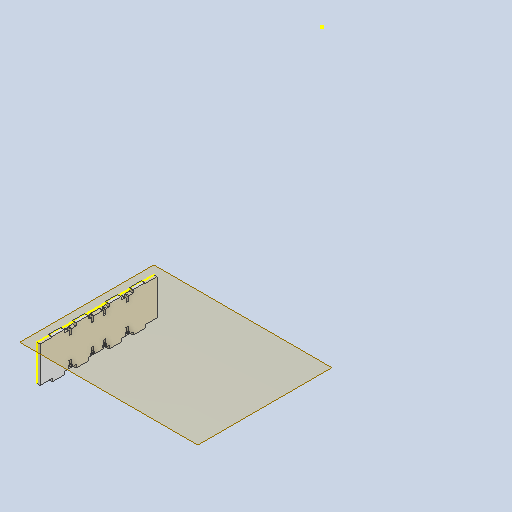
# Autodesk Inventor part: стенка
Saved by Autodesk Inventor 2024.2 (Build 282272000, 272)
## iProperties
Created: 2025-12-09
Part Number: стенка
Material: Типовые
Document SubType Name: Modeling
Designer: katya_notebook
Mass: 65.1748 g
Surface Area: 247.334 cm^2
Volume: 65.1748 cm^3
Density: 1 g/cm^3
Appearance: По умолчанию
Author: katya_notebook
Autodesk Inventor part; units mm, degrees
ref_plane "YZ Plane" through (0, 0, 0) normal (1, 0, 0) x (0, 1, 0)
ref_plane "XZ Plane" through (0, 0, 0) normal (0, 1, 0) x (-1, 0, 0)
ref_plane "XY Plane" through (0, 0, 0) normal (0, 0, 1) x (1, 0, 0)
ref_plane "РабПлоскость1" through (-475.2675, -216.9886, 379.0883) normal (0, 1, 0) x (-1, 0, 0)
sketch "Эскиз1" plane through (-475.2675, -216.9886, 379.0883) normal (0, 1, 0) x (-1, 0, 0)
  line L0 (135, 97.5) -> (129, 97.5)
  line L1 (129, 97.5) -> (129, -97.5)
  line L2 (129, -97.5) -> (135, -97.5)
  line L3 (135, -97.5) -> (135, 97.5)
  line L4 (135, -97.5) -> (135, 97.5) projected
  line L5 (127, 97.5) -> (62.5237, 97.5) projected
  line L6 (62.5237, -97.5) -> (127, -97.5) projected
  point P0 (-475.2675, -379.0883)
  dimension "d0" = 0
  dimension "d1" = 6
  dimension "d2" = 0
  dimension "d3" = 0
  constraints: 8 end point, 2 parallel, 1 horizontal, 1 perpendicular, 1 vertical alignment
  measures "d0" horizontal extent of L3
  measures "d1" distance of L0.start L0.end
  measures "d2" distance between parallel lines of L6 L2
  measures "d3" distance between parallel lines of L0 L5
ref_plane "РабПлоскость2" through (-610.2675, -276.6936, 277.5883) normal (0, 1, 0) x (0, 0, 1)
extrude "Выдавливание1" add sketch "Эскиз1" against normal up to surface (59.705 mm away)
sketch "Эскиз2" plane through (-610.2675, -216.9886, 281.5883) normal (-1, 0, 0) x (0, 0, 1)
  line L0 (175, -4) -> (187, -4) projected
  line L1 (195, 0) -> (195, -59.705) projected
  line L2 (0, 0) -> (195, 0) projected
  line L3 (0, 0) -> (0, -59.705) projected
  point P0 (-281.5883, 216.9886)
  point P1 (195, -59.705)
  point P2 (0, -59.705)
  constraints: 2 other
sketch "Эскиз3" plane through (-610.2675, -276.6936, 281.5883) normal (-1, 0, 0) x (0, 0, 1)
  line L0 (195, 0) -> (0, 0) projected
  line L1 (175, 0) -> (155, 0)
  line L2 (155, 0) -> (155, -5)
  line L3 (155, -5) -> (175, -5)
  line L4 (175, -5) -> (175, 0)
  line L5 (195, 59.705) -> (195, 0) projected
  line L6 (135, 0) -> (115, 0)
  line L7 (115, 0) -> (115, -5)
  line L8 (115, -5) -> (135, -5)
  line L9 (135, -5) -> (135, 0)
  line L10 (20, 0) -> (40, 0)
  line L11 (40, 0) -> (40, -5)
  line L12 (40, -5) -> (20, -5)
  line L13 (20, -5) -> (20, 0)
  line L14 (60, 0) -> (80, 0)
  line L15 (80, 0) -> (80, -5)
  line L16 (80, -5) -> (60, -5)
  line L17 (60, -5) -> (60, 0)
  line L18 (97.5, 27.8525) -> (226.4185, 27.8525)
  line L19 (195, 55.705) -> (0, 55.705)
  line L20 (175, 55.705) -> (155, 55.705)
  line L21 (155, 55.705) -> (155, 60.705)
  line L22 (155, 60.705) -> (175, 60.705)
  line L23 (175, 60.705) -> (175, 55.705)
  line L24 (135, 55.705) -> (115, 55.705)
  line L25 (115, 55.705) -> (115, 60.705)
  line L26 (115, 60.705) -> (135, 60.705)
  line L27 (135, 60.705) -> (135, 55.705)
  line L28 (20, 55.705) -> (40, 55.705)
  line L29 (40, 55.705) -> (40, 60.705)
  line L30 (40, 60.705) -> (20, 60.705)
  line L31 (20, 60.705) -> (20, 55.705)
  line L32 (60, 55.705) -> (80, 55.705)
  line L33 (80, 55.705) -> (80, 60.705)
  line L34 (80, 60.705) -> (60, 60.705)
  line L35 (60, 60.705) -> (60, 55.705)
  point P0 (-281.5883, 276.6936)
  point P1 (40, 55.705)
  point P2 (80, 55.705)
  point P3 (40, 0)
  point P4 (80, 0)
  point P5 (115, 55.705)
  point P6 (155, 55.705)
  point P7 (115, 0)
  point P8 (155, 0)
  dimension "d8" = 5
  dimension "d9" = 20
  dimension "d10" = 20
  dimension "d11" = 20
  dimension "d12" = 20
  dimension "d13" = 5
  dimension "d14" = 20
  dimension "d15" = 20
  dimension "d16" = 20
  dimension "d17" = 20
  dimension "d43" = 5
  constraints: 68 end point, 17 symmetric about line, 8 parallel, 8 point on line, 5 horizontal, 4 perpendicular
  measures "d8" distance of L3.end L1.start
  measures "d9" distance of L2.end L3.end
  measures "d10" distance of L0.start L1.start
  measures "d11" distance of L7.end L8.end
  measures "d12" distance of L1.end L6.start
  measures "d13" distance of L10.end L11.end
  measures "d14" distance of L11.end L12.end
  measures "d15" distance of L10.start L0.end
  measures "d16" distance of L15.end L16.end
  measures "d17" distance of L14.start L10.end
  measures "d43" distance of L16.end L14.start
extrude "Выдавливание3" add sketch "Эскиз3" against normal blind 6
sketch "Эскиз4" plane through (-610.2675, -276.6936, 281.5883) normal (-1, 0, 0) x (0, 0, 1)
  point P0 (-281.5883, 276.6936)
sketch "Эскиз5" plane through (-610.2675, -276.6936, 281.5883) normal (-1, 0, 0) x (0, 0, 1)
  point P0 (-281.5883, 276.6936)
sketch "Эскиз6" plane through (-610.2675, -276.6936, 281.5883) normal (-1, 0, 0) x (0, 0, 1)
  line L0 (111.125, 1.5) -> (104.625, 1.5)
  line L1 (104.625, 1.5) -> (104.625, 4.5)
  line L2 (104.625, 4.5) -> (111.125, 4.5)
  line L3 (111.125, 4.5) -> (111.125, 1.5)
  line L4 (115, 0) -> (115, -5) projected
  line L5 (90.375, 1.5) -> (83.875, 1.5)
  line L6 (83.875, 1.5) -> (83.875, 4.5)
  line L7 (83.875, 4.5) -> (90.375, 4.5)
  line L8 (90.375, 4.5) -> (90.375, 1.5)
  line L9 (111.125, 3) -> (104.625, 3)
  line L10 (115, 0) -> (80, 0) projected
  line L11 (106.125, 6) -> (109.625, 6)
  line L12 (109.625, 6) -> (109.625, 0)
  line L13 (109.625, 0) -> (106.125, 0)
  line L14 (106.125, 0) -> (106.125, 6)
  line L15 (106.125, 6) -> (109.625, 0) construction
  line L16 (109.625, 6) -> (106.125, 0) construction
  line L17 (90.375, 3) -> (83.875, 3)
  line L18 (87.125, 1.5) -> (87.125, 4.5)
  line L19 (85.375, 6) -> (88.875, 6)
  line L20 (88.875, 6) -> (88.875, 0)
  line L21 (88.875, 0) -> (85.375, 0)
  line L22 (85.375, 0) -> (85.375, 6)
  line L23 (85.375, 6) -> (88.875, 0) construction
  line L24 (88.875, 6) -> (85.375, 0) construction
  line L25 (148.25, 1.5) -> (141.75, 1.5)
  line L26 (141.75, 1.5) -> (141.75, 4.5)
  line L27 (141.75, 4.5) -> (148.25, 4.5)
  line L28 (148.25, 4.5) -> (148.25, 1.5)
  line L29 (148.25, 3) -> (141.75, 3)
  line L30 (143.25, 12) -> (146.75, 12)
  line L31 (146.75, 12) -> (146.75, -6)
  line L32 (146.75, -6) -> (143.25, -6)
  line L33 (143.25, -6) -> (143.25, 12)
  line L34 (143.25, 12) -> (146.75, -6) construction
  line L35 (146.75, 12) -> (143.25, -6) construction
  line L36 (155, 0) -> (155, -5) projected
  line L37 (53.25, 1.5) -> (46.75, 1.5)
  line L38 (46.75, 1.5) -> (46.75, 4.5)
  line L39 (46.75, 4.5) -> (53.25, 4.5)
  line L40 (53.25, 4.5) -> (53.25, 1.5)
  line L41 (53.25, 3) -> (46.75, 3)
  line L42 (48.25, 12) -> (51.75, 12)
  line L43 (51.75, 12) -> (51.75, -6)
  line L44 (51.75, -6) -> (48.25, -6)
  line L45 (48.25, -6) -> (48.25, 12)
  line L46 (48.25, 12) -> (51.75, -6) construction
  line L47 (51.75, 12) -> (48.25, -6) construction
  line L48 (60, 0) -> (60, -5) projected
  line L49 (195, 59.705) -> (195, 0) projected
  line L50 (195, 29.8525) -> (88.875, 29.8525)
  line L51 (111.125, 58.205) -> (104.625, 58.205)
  line L52 (104.625, 58.205) -> (104.625, 55.205)
  line L53 (104.625, 55.205) -> (111.125, 55.205)
  line L54 (111.125, 55.205) -> (111.125, 58.205)
  line L55 (115, 59.705) -> (115, 64.705)
  line L56 (90.375, 58.205) -> (83.875, 58.205)
  line L57 (83.875, 58.205) -> (83.875, 55.205)
  line L58 (83.875, 55.205) -> (90.375, 55.205)
  line L59 (90.375, 55.205) -> (90.375, 58.205)
  line L60 (111.125, 56.705) -> (104.625, 56.705)
  line L61 (115, 59.705) -> (80, 59.705)
  line L62 (106.125, 53.705) -> (109.625, 53.705)
  line L63 (109.625, 53.705) -> (109.625, 59.705)
  line L64 (109.625, 59.705) -> (106.125, 59.705)
  line L65 (106.125, 59.705) -> (106.125, 53.705)
  line L66 (106.125, 53.705) -> (109.625, 59.705) construction
  line L67 (109.625, 53.705) -> (106.125, 59.705) construction
  line L68 (90.375, 56.705) -> (83.875, 56.705)
  line L69 (87.125, 58.205) -> (87.125, 55.205)
  line L70 (85.375, 53.705) -> (88.875, 53.705)
  line L71 (88.875, 53.705) -> (88.875, 59.705)
  line L72 (88.875, 59.705) -> (85.375, 59.705)
  line L73 (85.375, 59.705) -> (85.375, 53.705)
  line L74 (85.375, 53.705) -> (88.875, 59.705) construction
  line L75 (88.875, 53.705) -> (85.375, 59.705) construction
  line L76 (146.75, 65.705) -> (143.25, 65.705)
  line L77 (146.75, 47.705) -> (146.75, 65.705)
  line L78 (146.75, 47.705) -> (143.25, 65.705) construction
  line L79 (143.25, 47.705) -> (146.75, 65.705) construction
  line L80 (143.25, 65.705) -> (143.25, 47.705)
  line L81 (141.75, 58.205) -> (141.75, 55.205)
  line L82 (148.25, 58.205) -> (141.75, 58.205)
  line L83 (148.25, 55.205) -> (148.25, 58.205)
  line L84 (141.75, 55.205) -> (148.25, 55.205)
  line L85 (148.25, 56.705) -> (141.75, 56.705)
  line L86 (143.25, 47.705) -> (146.75, 47.705)
  line L87 (155, 59.705) -> (155, 64.705)
  line L88 (51.75, 65.705) -> (48.25, 65.705)
  line L89 (51.75, 47.705) -> (51.75, 65.705)
  line L90 (51.75, 47.705) -> (48.25, 65.705) construction
  line L91 (48.25, 47.705) -> (51.75, 65.705) construction
  line L92 (48.25, 65.705) -> (48.25, 47.705)
  line L93 (46.75, 58.205) -> (46.75, 55.205)
  line L94 (53.25, 58.205) -> (46.75, 58.205)
  line L95 (53.25, 55.205) -> (53.25, 58.205)
  line L96 (46.75, 55.205) -> (53.25, 55.205)
  line L97 (53.25, 56.705) -> (46.75, 56.705)
  line L98 (48.25, 47.705) -> (51.75, 47.705)
  line L99 (60, 59.705) -> (60, 64.705)
  line L100 (109.625, 6) -> (106.125, 6)
  line L101 (106.125, 6) -> (106.125, 12)
  line L102 (106.125, 12) -> (109.625, 12)
  line L103 (109.625, 12) -> (109.625, 6)
  line L104 (88.875, 6) -> (85.375, 6)
  line L105 (85.375, 6) -> (85.375, 12)
  line L106 (85.375, 12) -> (88.875, 12)
  line L107 (88.875, 12) -> (88.875, 6)
  line L108 (109.625, 53.705) -> (106.125, 53.705)
  line L109 (106.125, 53.705) -> (106.125, 47.705)
  line L110 (106.125, 47.705) -> (109.625, 47.705)
  line L111 (109.625, 47.705) -> (109.625, 53.705)
  line L112 (88.875, 53.705) -> (85.375, 53.705)
  line L113 (85.375, 53.705) -> (85.375, 47.705)
  line L114 (85.375, 47.705) -> (88.875, 47.705)
  line L115 (88.875, 47.705) -> (88.875, 53.705)
  point P0 (-281.5883, 276.6936)
  point P1 (115, -2.5)
  point P2 (107.875, 11.6549)
  point P3 (107.875, 3)
  point P4 (99.25, 0)
  point P5 (87.125, 3)
  point P6 (149.0518, 14.6563)
  point P7 (145, 3)
  point P8 (155, -2.5)
  point P9 (49.2049, 25.9501)
  point P10 (50, 3)
  point P11 (60, -2.5)
  point P12 (48.25, 4.5)
  point P13 (48.25, 1.5)
  point P14 (51.75, 1.5)
  point P15 (51.75, 4.5)
  point P16 (88.875, 4.5)
  point P17 (85.375, 4.5)
  point P18 (85.375, 1.5)
  point P19 (85.375, 0)
  point P20 (88.875, 1.5)
  point P21 (106.125, 1.5)
  point P22 (106.125, 0)
  point P23 (109.625, 1.5)
  point P24 (109.625, 4.5)
  point P25 (106.125, 4.5)
  point P26 (143.25, 1.5)
  point P27 (146.75, 1.5)
  point P28 (146.75, 4.5)
  point P29 (143.25, 4.5)
  point P30 (195, 55.705)
  point P31 (115, 62.205)
  point P32 (107.875, 48.0501)
  point P33 (107.875, 56.705)
  point P34 (99.25, 59.705)
  point P35 (87.125, 56.705)
  point P36 (145, 56.705)
  point P37 (149.0518, 45.0486)
  point P38 (155, 62.205)
  point P39 (50, 56.705)
  point P40 (60, 62.205)
  point P41 (51.75, 55.205)
  point P42 (51.75, 58.205)
  point P43 (48.25, 58.205)
  point P44 (48.25, 55.205)
  point P45 (88.875, 55.205)
  point P46 (88.875, 58.205)
  point P47 (85.375, 55.705)
  point P48 (85.375, 58.205)
  point P49 (85.375, 55.205)
  point P50 (106.125, 58.205)
  point P51 (106.125, 55.205)
  point P52 (109.625, 55.205)
  point P53 (109.625, 58.205)
  point P54 (143.25, 58.205)
  point P55 (143.25, 55.205)
  point P56 (146.75, 55.205)
  point P57 (146.75, 58.205)
  point P58 (85.375, 59.705)
  point P59 (85.375, 53.705)
  point P60 (106.125, 53.705)
  point P61 (85.375, 6)
  point P62 (106.125, 6)
  point P63 (85.375, 0)
  point P64 (85.375, 59.705)
  point P65 (85.375, 53.705)
  point P66 (85.375, 6)
  dimension "d1" = 6
  dimension "d20" = 6.5
  dimension "d21" = 3
  dimension "d22" = 3.875
  dimension "d26" = 6.5
  dimension "d27" = 3
  dimension "d29" = 3
  dimension "d30" = 3.5
  dimension "d32" = 3.5
  dimension "d33" = 6.5
  dimension "d34" = 3
  dimension "d35" = 3.5
  dimension "d36" = 8.25
  dimension "d37" = 6.5
  dimension "d38" = 3
  dimension "d39" = 3.5
  dimension "d40" = 8.25
  dimension "d46" = 6
  dimension "d47" = 6
  constraints: 222 end point, 59 symmetric about line, 26 midpoint, 24 parallel, 13 horizontal, 13 perpendicular, 6 point on line, 5 collinear
  measures "d20" distance of L0.start L0.end
  measures "d21" distance of L0.end L1.end
  measures "d22" horizontal distance of L9.start point (115, -2.5)
  measures "d26" distance of L5.start L5.end
  measures "d27" distance of L5.end L6.end
  measures "d29" distance from line of L10 point (107.875, 3)
  measures "d30" distance of L12.end L13.end
  measures "d32" distance of L21.end L20.end
  measures "d33" distance of L25.start L26.start
  measures "d34" distance of L26.start L26.end
  measures "d35" distance of L32.start L32.end
  measures "d36" distance from line of L31 point (155, -2.5)
  measures "d37" distance of L37.start L38.start
  measures "d38" distance of L38.start L38.end
  measures "d39" distance of L44.start L44.end
  measures "d40" distance from line of L43 point (60, -2.5)
  measures "d46" distance of L100.end L101.end
  measures "d47" distance of L108.end L109.end
extrude "Выдавливание4" cut sketch "Эскиз6" against normal blind 6
sketch "Эскиз7" plane through (-610.2675, -276.6936, 281.5883) normal (-1, 0, 0) x (0, 0, 1)
  line L0 (175, 55.705) -> (187, 55.705) projected
  line L1 (195, 59.705) -> (195, 0) projected
  line L2 (175, 59.705) -> (195, 59.705) projected
  line L3 (175, 59.705) -> (175, 55.705) projected
  line L4 (155, 55.705) -> (155, 59.705) projected
  line L5 (135, 55.705) -> (155, 55.705) projected
  line L6 (135, 59.705) -> (135, 55.705) projected
  line L7 (135, 59.705) -> (155, 59.705) projected
  line L8 (80, 55.705) -> (115, 55.705) projected
  line L9 (115, 55.705) -> (115, 59.705) projected
  line L10 (80, 59.705) -> (80, 55.705) projected
  line L11 (80, 59.705) -> (115, 59.705) projected
  line L12 (60, 55.705) -> (60, 59.705) projected
  line L13 (40, 55.705) -> (60, 55.705) projected
  line L14 (40, 59.705) -> (60, 59.705) projected
  line L15 (40, 59.705) -> (40, 55.705) projected
  line L16 (175, 55.705) -> (20, 55.705) projected
  line L17 (20, 55.705) -> (20, 59.705) projected
  line L18 (0, 59.705) -> (20, 59.705) projected
  line L19 (0, 59.705) -> (0, 0) projected
  point P0 (-281.5883, 276.6936)
  point P1 (195, 0)
  point P2 (0, 0)
  point P3 (175, 59.705)
  constraints: 2 other
extrude "Выдавливание5" cut sketch "Эскиз7" against normal blind 6
